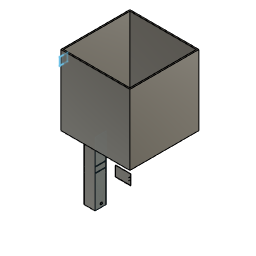
eis v2 (Autodesk Fusion 360 design; units mm, degrees)
Autodesk Fusion 360 part; units mm, degrees
sketch "Skizze1" plane through (0, 0, 0) normal (1, 0, 0) x (0, 1, 0)
  line L0 (-14.6111, 11.8997) -> (15.3889, 11.8997)
  line L1 (15.3889, 11.8997) -> (15.3889, -18.1003)
  line L2 (15.3889, -18.1003) -> (-14.6111, -18.1003)
  line L3 (-14.6111, -18.1003) -> (-14.6111, 11.8997)
  dimension "d1" = 30
  dimension "d2" = 30
  constraint horizontal L0
  constraint vertical L1
  constraint horizontal L2
  constraint vertical L3
  measures "d1" distance of L0.start L0.end
  measures "d2" distance of L0.start L2.end
sketch "Skizze2" plane through (0, 0, 0) normal (0, 1, 0) x (1, 0, 0)
  line L0 (-10, -25) -> (260, -25)
  line L1 (260, -25) -> (260, 245)
  line L2 (260, 245) -> (-10, 245)
  line L3 (-10, 245) -> (-10, -25)
  dimension "d3" = 270
  dimension "d4" = 270
  constraint horizontal L0
  constraint vertical L1
  constraint horizontal L2
  constraint vertical L3
  measures "d3" distance of L0.start L0.end
  measures "d4" distance of L0.start L2.end
extrude "Extrusion1" add sketch "Skizze2" along normal blind 270 makes body 1
shell "Schale1" thickness 5 removed faces 1 at (80, 90, 25) on bodies 1
extrude "Extrusion2" add 1 faces at (170, 90, -245) along direction (0, 0, -1) blind 5 on bodies 1 bodies 1
sketch "Skizze3" plane through (0, 0, -240) normal (0, 0, 1) x (-1, 0, 0)
  line L0 (5, -5) -> (-255, -5)
  line L1 (-255, -5) -> (-255, -265)
  line L2 (-255, -265) -> (5, -265)
  line L3 (5, -265) -> (5, -5)
  line L4 (-77.069, -46.694) -> (-37.069, -46.694)
  line L5 (-37.069, -46.694) -> (-37.069, -86.694)
  line L6 (-37.069, -86.694) -> (-77.069, -86.694)
  line L7 (-77.069, -86.694) -> (-77.069, -46.694)
  dimension "d10" = 40
  dimension "d11" = 40
  constraint horizontal L4
  constraint vertical L5
  constraint horizontal L6
  constraint vertical L7
  measures "d10" distance of L4.start L4.end
  measures "d11" distance of L4.end L5.end
extrude "Extrusion3" cut sketch "Skizze3" against normal blind 230 contours L4 L5 L6 L7 bodies 1
fillet "Abrundung1" radius 90 4 edges at (37.069, 66.694, -240) (57.069, 86.694, -240) (77.069, 66.694, -240) (57.069, 46.694, -240) on bodies 1
sketch "Skizze4" plane through (0, 0, -250) normal (0, 0, -1) x (1, 0, 0)
  line L0 (37.069, -86.694) -> (37.069, -46.694)
  line L1 (37.069, -46.694) -> (77.069, -46.694)
  line L2 (77.069, -46.694) -> (77.069, -86.694)
  line L3 (77.069, -86.694) -> (37.069, -86.694)
  line L4 (260, 0) -> (-10, 0)
  line L5 (-10, 0) -> (-10, -270)
  line L6 (-10, -270) -> (260, -270)
  line L7 (260, -270) -> (260, 0)
  line L8 (32.069, -41.694) -> (82.069, -41.694)
  line L9 (82.069, -41.694) -> (82.069, -91.694)
  line L10 (82.069, -91.694) -> (32.069, -91.694)
  line L11 (32.069, -91.694) -> (32.069, -41.694)
  dimension "d16" = 5
  dimension "d17" = 5
  dimension "d18" = 5
  dimension "d19" = 5
  constraint horizontal L8
  constraint vertical L9
  constraint horizontal L10
  constraint vertical L11
  measures "d16" distance of L1 L8
  measures "d17" distance of L0 L11
  measures "d18" distance of L3 L10
  measures "d19" distance of L2 L9
extrude "Extrusion4" add sketch "Skizze4" along normal blind 50 contours L8 L9 L10 L11 bodies 1
extrude "Extrusion5" add 1 faces at (63.7357, 90.0273, -300) along direction (0, 0, -1) blind 200 on bodies 1 bodies 1
sketch "Skizze5" plane through (82.069, 0, 0) normal (1, 0, 0) x (0, 1, 0)
  line L0 (91.694, -250) -> (41.694, -250)
  line L1 (41.694, -250) -> (41.694, -500)
  line L2 (41.694, -500) -> (91.694, -500)
  line L3 (91.694, -500) -> (91.694, -250)
  line L4 (86.694, -350) -> (46.694, -350)
  line L5 (46.694, -350) -> (46.694, -352)
  line L6 (46.694, -352) -> (86.694, -352)
  line L7 (86.694, -352) -> (86.694, -350)
  line L8 (86.694, -372) -> (46.694, -372)
  line L9 (46.694, -372) -> (46.694, -374)
  line L10 (46.694, -374) -> (86.694, -374)
  line L11 (86.694, -374) -> (86.694, -372)
  dimension "d24" = 20
  dimension "d25" = 5
  dimension "d26" = 5
  dimension "d27" = 5
  dimension "d28" = 5
  dimension "d29" = 2
  dimension "d30" = 2
  dimension "d31" = 100
  constraint horizontal L4
  constraint vertical L5
  constraint horizontal L6
  constraint vertical L7
  constraint horizontal L8
  constraint vertical L9
  constraint horizontal L10
  constraint vertical L11
  measures "d24" distance of L6 L8
  measures "d25" distance of L3 L11
  measures "d26" distance of L3 L7
  measures "d27" distance of L1 L5
  measures "d28" distance of L1 L9
  measures "d29" distance of L8.start L10.end
  measures "d30" distance of L4.start L6.end
  measures "d31" distance of L0 L4
extrude "Extrusion6" cut sketch "Skizze5" against normal blind 10 contours L4 L5 L6 L7 | L8 L9 L10 L11 bodies 1
extrude "Extrusion7" cut 1 faces at (82.069, 73.3606, -458) along direction (-1, 0, 0) blind 3 on bodies 1 bodies 1
extrude "Extrusion8" cut 1 faces at (49.4023, 91.694, -416.6667) along direction (0, -1, 0) blind 3 on bodies 1 bodies 1
extrude "Extrusion9" cut 1 faces at (32.069, 73.0273, -333.3333) along direction (1, 0, 0) blind 3 on bodies 1 bodies 1
extrude "Extrusion10" cut 1 faces at (49.7357, 41.694, -333.3333) along direction (0, 1, 0) blind 3 on bodies 1 bodies 1
sketch "Skizze6" plane through (35.069, 0, 0) normal (-1, 0, 0) x (0, -1, 0)
  line L0 (-44.694, -500) -> (-44.694, -250)
  line L1 (-44.694, -250) -> (-88.694, -250)
  line L2 (-88.694, -250) -> (-88.694, -500)
  line L3 (-88.694, -500) -> (-44.694, -500)
  line L4 (-86.694, -370) -> (-46.694, -370)
  line L5 (-46.694, -370) -> (-46.694, -372)
  line L6 (-46.694, -372) -> (-86.694, -372)
  line L7 (-86.694, -372) -> (-86.694, -370)
  line L8 (-86.694, -392) -> (-46.694, -392)
  line L9 (-46.694, -392) -> (-46.694, -394)
  line L10 (-46.694, -394) -> (-86.694, -394)
  line L11 (-86.694, -394) -> (-86.694, -392)
  dimension "d42" = 2
  dimension "d43" = 2
  dimension "d44" = 2
  dimension "d45" = 2
  dimension "d46" = 2
  dimension "d47" = 2
  dimension "d48" = 20
  dimension "d49" = 120
  constraint horizontal L4
  constraint vertical L5
  constraint horizontal L6
  constraint vertical L7
  constraint horizontal L8
  constraint vertical L9
  constraint horizontal L10
  constraint vertical L11
  measures "d42" distance of L2 L7
  measures "d43" distance of L2 L11
  measures "d44" distance of L0 L5
  measures "d45" distance of L0 L9
  measures "d46" distance of L8 L10
  measures "d47" distance of L4 L6
  measures "d48" distance of L6 L8
  measures "d49" distance of L1 L4
extrude "Extrusion11" cut sketch "Skizze6" against normal blind 2 contours L4 L5 L6 L7 | L8 L9 L10 L11 bodies 1
sketch "Skizze7" plane through (79.069, 0, 0) normal (1, 0, 0) x (0, 1, 0)
  line L0 (46.694, -372) -> (86.694, -372)
  line L1 (86.694, -372) -> (86.694, -374)
  line L2 (86.694, -374) -> (46.694, -374)
  line L3 (46.694, -374) -> (46.694, -372)
  line L4 (46.694, -350) -> (86.694, -350)
  line L5 (86.694, -350) -> (86.694, -352)
  line L6 (86.694, -352) -> (46.694, -352)
  line L7 (46.694, -352) -> (46.694, -350)
  line L8 (44.694, -250) -> (44.694, -500)
  line L9 (44.694, -500) -> (88.694, -500)
  line L10 (88.694, -500) -> (88.694, -250)
  line L11 (88.694, -250) -> (44.694, -250)
hole "Bohrung1" at (79.069, 69.3254, -487.0132) direction (-1, 0, 0) diameter 9 depth 5 tip angle 118 bodies 1
sketch "Skizze8" plane through (0, 44.694, 0) normal (0, -1, 0) x (1, 0, 0)
  line L0 (35.069, -250) -> (35.069, -500)
  line L1 (35.069, -500) -> (79.069, -500)
  line L2 (79.069, -500) -> (79.069, -250)
  line L3 (79.069, -250) -> (35.069, -250)
  line L4 (159.1989, -304.3397) -> (219.1989, -304.3397)
  line L5 (219.1989, -304.3397) -> (219.1989, -344.3397)
  line L6 (219.1989, -344.3397) -> (159.1989, -344.3397)
  line L7 (159.1989, -344.3397) -> (159.1989, -304.3397)
  dimension "d55" = 60
  dimension "d56" = 40
  constraint horizontal L4
  constraint vertical L5
  constraint horizontal L6
  constraint vertical L7
  measures "d55" distance of L4.start L4.end
  measures "d56" distance of L4.start L6.end
extrude "Extrusion12" add sketch "Skizze8" along normal blind 1 separate body contours L4 L5 L6 L7 makes body 2
sketch "Skizze9" plane through (0, 43.694, 0) normal (0, -1, 0) x (1, 0, 0)
  line L0 (159.1989, -344.3397) -> (219.1989, -344.3397)
  line L1 (219.1989, -344.3397) -> (219.1989, -304.3397)
  line L2 (219.1989, -304.3397) -> (159.1989, -304.3397)
  line L3 (159.1989, -304.3397) -> (159.1989, -344.3397)
  circle A0 centre (213.1989, -319.3397) radius 1.5
  circle A1 centre (213.1989, -329.3397) radius 1.5
  dimension "d59" = 3
  dimension "d60" = 3
  dimension "d61" = 6
  dimension "d62" = 6
  dimension "d63" = 15
  dimension "d64" = 15
  measures "d59" diameter of A0
  measures "d60" diameter of A1
  measures "d61" distance of L1 A1.centre
  measures "d62" distance of L1 A0.centre
  measures "d63" distance of L0 A1.centre
  measures "d64" distance of L2 A0.centre
extrude "Extrusion13" cut sketch "Skizze9" against normal blind 5 contours A0 | A1 bodies 2
